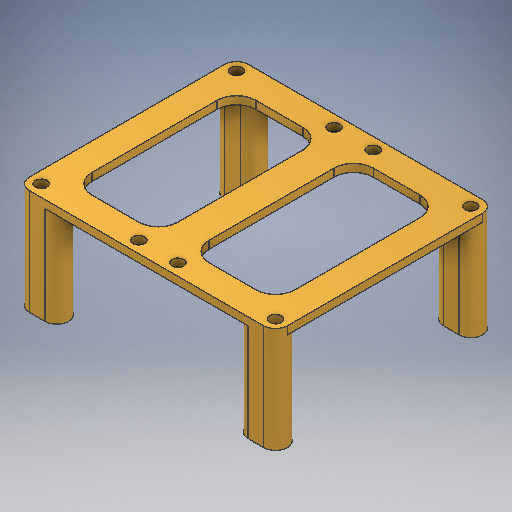
# Autodesk Inventor part: electronics_holder
Saved by Autodesk Inventor 2026.1 (Build 301233000, 233)
## iProperties
Created: 2025-12-21
Part Number: electronics_holder
Material: Generic
Document SubType Name: Modeling
Designer: emanuel
Density: 1 g/cm^3
Appearance: Default
Author: emanuel
Autodesk Inventor part; units mm, degrees
ref_plane "YZ Plane" through (0, 0, 0) normal (1, 0, 0) x (0, 1, 0)
ref_plane "XZ Plane" through (0, 0, 0) normal (0, 1, 0) x (-1, 0, 0)
ref_plane "XY Plane" through (0, 0, 0) normal (0, 0, 1) x (1, 0, 0)
sketch "Sketch1" plane through (0, 0, 0) normal (0, 1, 0) x (-1, 0, 0)
  line L0 (0, 0) -> (60, 0)
  line L1 (60, 0) -> (60, -50)
  line L2 (60, -50) -> (0, -50)
  line L3 (0, -50) -> (0, 0)
  line L4 (0, 0) -> (7, 0)
  circle A0 centre (0, 0) radius 1.5
  circle A1 centre (60, 0) radius 1.5
  circle A2 centre (60, -50) radius 1.5
  circle A3 centre (0, -50) radius 1.5
  line L5 (60, -50) -> (53, -50)
  line L6 (7, 0) -> (53, 0)
  line L7 (53, 0) -> (53, -50)
  line L8 (53, -50) -> (7, -50)
  line L9 (7, -50) -> (7, 0)
  line L10 (60, 0) -> (63, 0)
  line L11 (63, 0) -> (63, 3)
  line L12 (63, 3) -> (60, 3)
  line L13 (60, 3) -> (60, 0)
  line L14 (0, -50) -> (-3, -50)
  line L15 (-3, -50) -> (-3, -53)
  line L16 (-3, -53) -> (0, -53)
  line L17 (0, -53) -> (0, -50)
  line L18 (-3, -53) -> (63, -53)
  line L19 (63, -53) -> (63, 3)
  line L20 (63, 3) -> (-3, 3)
  line L21 (-3, 3) -> (-3, -53)
  line L22 (63, -53) -> (53, -53)
  line L23 (53, -53) -> (53, -47)
  line L24 (53, -47) -> (63, -47)
  line L25 (63, -47) -> (63, -53)
  line L26 (-3, -53) -> (7, -53)
  line L27 (7, -53) -> (7, -47)
  line L28 (7, -47) -> (-3, -47)
  line L29 (-3, -47) -> (-3, -53)
  line L30 (-3, 3) -> (7, 3)
  line L31 (7, 3) -> (7, -3)
  line L32 (7, -3) -> (-3, -3)
  line L33 (-3, -3) -> (-3, 3)
  line L34 (63, 3) -> (53, 3)
  line L35 (53, 3) -> (53, -3)
  line L36 (53, -3) -> (63, -3)
  line L37 (63, -3) -> (63, 3)
  point P0 (7, 3)
  point P1 (-3, -3)
  point P2 (7, -53)
  point P3 (7, -50)
  point P4 (-3, -47)
  dimension "d0" = 60
  dimension "d1" = 50
  dimension "d2" = 7
  dimension "d3" = 3
  dimension "d4" = 3
  dimension "d5" = 3
  dimension "d6" = 3
  dimension "d7" = 7
  dimension "d8" = 3
  dimension "d9" = 3
  dimension "d10" = 3
  dimension "d11" = 3
  dimension "d12" = 6
  dimension "d13" = 6
  dimension "d14" = 6
  dimension "d15" = 6
  constraints: 76 end point, 18 parallel, 9 horizontal, 9 perpendicular, 6 point on line, 4 centre point, 4 coincident
  measures "d0" distance of L1.end L2.end
  measures "d1" distance of L0.end L1.end
  measures "d2" distance of L0.start L4.end
  measures "d3" diameter of A0
  measures "d4" diameter of A1
  measures "d5" diameter of A2
  measures "d6" diameter of A3
  measures "d7" distance of L5.start L5.end
  measures "d8" distance of L12.end L11.end
  measures "d9" distance of L11.end L10.end
  measures "d10" distance of L16.end L15.end
  measures "d11" distance of L15.end L14.end
  measures "d12" distance of L22.end L23.end
  measures "d13" distance of L27.end L26.end
  measures "d14" distance of L30.end L31.end
  measures "d15" distance of L35.end L34.end
extrude "Extrusion1" add sketch "Sketch1" along normal blind 2 contours A0 L3 L32 L21 L20 L31 L0 | L0 L9 L32 L3 A0 | L31 L20 L35 L0 | L0 L7 L2 L9 | L32 L9 L28 L3 | L3 L28 L21 L32 | L35 L20 L13 A1 L0 | L0 A1 L1 L36 L7 | L28 L9 L2 A3 L3 | L3 A3 L14 L21 L28 | L36 L1 L24 L7 | L13 L12 L11 L10 A1 | A1 L10 L19 L36 L1 | L24 L1 A2 L2 L7 | L36 L19 L24 L1 | L27 L18 L17 A3 L2 | L2 L23 L18 L27 | A3 L17 L16 L15 L14 | L2 A2 L1 L24 L19 L18 L23
extrude "Extrusion2" add sketch "Sketch1" against normal blind 25 contours A0 L3 L32 L21 L20 L31 L0 | L0 L9 L32 L3 A0 | L35 L20 L13 A1 L0 | L0 A1 L1 L36 L7 | L28 L9 L2 A3 L3 | L3 A3 L14 L21 L28 | L13 L12 L11 L10 A1 | A1 L10 L19 L36 L1 | L24 L1 A2 L2 L7 | L27 L18 L17 A3 L2 | A3 L17 L16 L15 L14 | L2 A2 L1 L24 L19 L18 L23
fillet "Fillet1" radius 3 16 edges at (3, -11.5, 3) (3, -12.5, -3) (-7, -12.5, 3) (-7, -12.5, -3) (3, -12.5, -47) (3, -11.5, -53) (-7, -12.5, -47) (-7, -12.5, -53) (-53, -12.5, -47) (-53, -12.5, -53) (-63, -12.5, -47) (-63, -11.5, -53) (-53, -12.5, 3) (-53, -12.5, -3) (-63, -11.5, 3) (-63, -12.5, -3)
sketch "Sketch2" plane through (0, -25, 0) normal (0, -1, 0) x (1, 0, 0)
  circle A0 centre (-60, 0) radius 1.5 projected
  arc A1 (-56, -3) -> (-56, 3) centre (-56, 0) ccw projected
  line L0 (-60, 0) -> (-56, 0)
  circle A2 centre (-56, 0) radius 1.5
  arc A3 (-4, 3) -> (-4, -3) centre (-4, 0) ccw projected
  circle A4 centre (-4, 0) radius 1.5
  arc A5 (-56, -53) -> (-56, -47) centre (-56, -50) ccw projected
  circle A6 centre (-56, -50) radius 1.5
  arc A7 (-4, -47) -> (-4, -53) centre (-4, -50) ccw projected
  circle A8 centre (-4, -50) radius 1.5
  point P0 (0, 0)
  dimension "d21" = 3
  dimension "d22" = 3
  dimension "d23" = 3
  dimension "d24" = 3
  constraints: 4 centre point, 4 coincident, 2 end point, 1 horizontal
  measures "d21" diameter of A2
  measures "d22" diameter of A4
  measures "d23" diameter of A6
  measures "d24" diameter of A8
extrude "Extrusion3" cut sketch "Sketch2" against normal blind 20 contours A2 | A4 | A6 | A8
sketch "Sketch4" plane through (0, 2, 0) normal (0, 1, 0) x (1, 0, 0)
  circle A0 centre (-60, 50) radius 1.5 projected
  circle A1 centre (0, 50) radius 1.5 projected
  line L0 (-60, 50) -> (0, 50)
  circle A2 centre (-60, 0) radius 1.5 projected
  circle A3 centre (0, 0) radius 1.5 projected
  line L1 (-60, 0) -> (0, 0)
  line L2 (-30, 50) -> (-30, 0)
  line L3 (-35, 0) -> (-25, 0)
  line L4 (-25, 0) -> (-25, 50)
  line L5 (-25, 50) -> (-35, 50)
  line L6 (-35, 50) -> (-35, 0)
  line L7 (-35, 0) -> (-25, 50) construction
  line L8 (-25, 0) -> (-35, 50) construction
  circle A4 centre (-35, 50) radius 1.5
  circle A5 centre (-25, 50) radius 1.5
  circle A6 centre (-35, 0) radius 1.5
  circle A7 centre (-25, 0) radius 1.5
  point P0 (-30, 25)
  dimension "d42" = 10
  dimension "d43" = 3
  dimension "d44" = 3
  dimension "d45" = 3
  dimension "d46" = 3
  constraints: 18 end point, 5 midpoint, 4 centre point, 4 coincident, 3 horizontal, 2 parallel, 1 perpendicular, 1 point on line
  measures "d42" distance of L5.end L4.end
  measures "d43" diameter of A4
  measures "d44" diameter of A5
  measures "d45" diameter of A6
  measures "d46" diameter of A7
extrude "Extrusion5" cut sketch "Sketch4" against normal blind 2 contours L0 A4 | L6 A4 L0 | L0 A4 L6 | A6 L1 L6 | L6 L1 A6 | A5 L0 | L0 L4 A5 | L1 A6 | L0 A5 L4 | A7 L4 L1 | L1 A7 | A7 L1 L4
sketch "Sketch5" plane through (0, 2, 0) normal (0, 1, 0) x (1, 0, 0)
  circle A0 centre (0, 50) radius 1.5 projected
  line L0 (0, 50) -> (-4, 50)
  line L1 (-4, 50) -> (-4, 46)
  line L2 (-4, 46) -> (0, 46)
  line L3 (0, 46) -> (0, 50)
  line L4 (0, 0) -> (-4, 0)
  line L5 (-4, 0) -> (-4, 4)
  line L6 (-4, 4) -> (0, 4)
  line L7 (0, 4) -> (0, 0)
  circle A1 centre (-60, 0) radius 1.5 projected
  line L8 (-60, 0) -> (-56, 0)
  line L9 (-56, 0) -> (-56, 4)
  line L10 (-56, 4) -> (-60, 4)
  line L11 (-60, 4) -> (-60, 0)
  line L12 (-56, 4) -> (-4, 4)
  line L13 (-4, 4) -> (-4, 46)
  line L14 (-4, 46) -> (-56, 46)
  line L15 (-56, 46) -> (-56, 4)
  line L16 (-30, 46) -> (-34, 46)
  line L17 (-34, 46) -> (-34, 4)
  line L18 (-34, 4) -> (-30, 4)
  line L19 (-30, 4) -> (-30, 46)
  line L20 (-30, 46) -> (-26, 46)
  line L21 (-26, 46) -> (-26, 4)
  line L22 (-26, 4) -> (-30, 4)
  line L23 (-30, 4) -> (-30, 46)
  dimension "d49" = 4
  dimension "d50" = 4
  dimension "d51" = 4
  dimension "d52" = 4
  dimension "d53" = 4
  dimension "d54" = 4
  dimension "d55" = 4
  dimension "d56" = 4
  constraints: 48 end point, 12 parallel, 6 horizontal, 6 perpendicular, 2 point on line, 1 midpoint
  measures "d49" distance of L2.end L1.end
  measures "d50" distance of L1.end L0.end
  measures "d51" distance of L5.end L6.end
  measures "d52" distance of L4.end L5.end
  measures "d53" distance of L10.end L9.end
  measures "d54" distance of L9.end L8.end
  measures "d55" distance of L18.end L17.end
  measures "d56" distance of L21.end L22.end
extrude "Extrusion6" cut sketch "Sketch5" against normal blind 2 contours L13 L12 L21 L14 | L17 L12 L15 L14
fillet "Fillet2" radius 5 8 edges at (-56, 1, -46) (-34, 1, -46) (-26, 1, -46) (-4, 1, -46) (-4, 1, -4) (-26, 1, -4) (-34, 1, -4) (-56, 1, -4)
body "Solid1"
